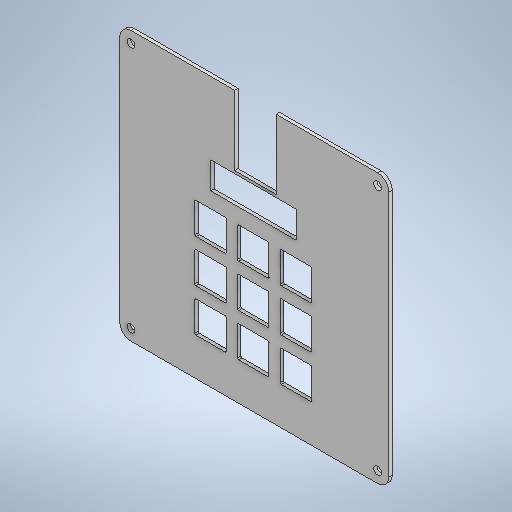
# Autodesk Inventor part: Top_Case_New
Saved by Autodesk Inventor 2025.1 (Build 291241000, 241)
## iProperties
Created: 2025-12-17
Part Number: Top_Case_New
Material: Generic
Document SubType Name: Modeling
Designer: omara
Density: 1 g/cm^3
Appearance: Default
Autodesk Inventor part; units mm, degrees
ref_plane "YZ Plane" through (0, 0, 0) normal (1, 0, 0) x (0, 1, 0)
ref_plane "XZ Plane" through (0, 0, 0) normal (0, 1, 0) x (-1, 0, 0)
ref_plane "XY Plane" through (0, 0, 0) normal (0, 0, 1) x (1, 0, 0)
sketch "Sketch1" plane through (0, 0, 0) normal (0, 0, 1) x (1, 0, 0)
  point P0 (0, 0)
sketch "0" plane through (0, 0, 0) normal (0, 0, 1) x (1, 0, 0)
  line L0 (3.025, -2.525) -> (16.025, -2.525)
  line L1 (3.025, -16.525) -> (16.025, -16.525)
  line L2 (2.525, -3.025) -> (2.525, -16.025)
  line L3 (16.525, -3.025) -> (16.525, -16.025)
  arc A0 (3.025, -2.525) -> (2.525, -3.025) centre (3.025, -3.025) ccw
  arc A1 (16.525, -3.025) -> (16.025, -2.525) centre (16.025, -3.025) ccw
  arc A2 (2.525, -16.025) -> (3.025, -16.525) centre (3.025, -16.025) ccw
  arc A3 (16.025, -16.525) -> (16.525, -16.025) centre (16.025, -16.025) ccw
  line L4 (22.075, -2.525) -> (35.075, -2.525)
  line L5 (22.075, -16.525) -> (35.075, -16.525)
  line L6 (21.575, -3.025) -> (21.575, -16.025)
  line L7 (35.575, -3.025) -> (35.575, -16.025)
  arc A4 (22.075, -2.525) -> (21.575, -3.025) centre (22.075, -3.025) ccw
  arc A5 (35.575, -3.025) -> (35.075, -2.525) centre (35.075, -3.025) ccw
  arc A6 (21.575, -16.025) -> (22.075, -16.525) centre (22.075, -16.025) ccw
  arc A7 (35.075, -16.525) -> (35.575, -16.025) centre (35.075, -16.025) ccw
  line L8 (41.125, -2.525) -> (54.125, -2.525)
  line L9 (41.125, -16.525) -> (54.125, -16.525)
  line L10 (40.625, -3.025) -> (40.625, -16.025)
  line L11 (54.625, -3.025) -> (54.625, -16.025)
  arc A8 (41.125, -2.525) -> (40.625, -3.025) centre (41.125, -3.025) ccw
  arc A9 (54.625, -3.025) -> (54.125, -2.525) centre (54.125, -3.025) ccw
  arc A10 (40.625, -16.025) -> (41.125, -16.525) centre (41.125, -16.025) ccw
  arc A11 (54.125, -16.525) -> (54.625, -16.025) centre (54.125, -16.025) ccw
  line L12 (3.025, -21.575) -> (16.025, -21.575)
  line L13 (3.025, -35.575) -> (16.025, -35.575)
  line L14 (2.525, -22.075) -> (2.525, -35.075)
  line L15 (16.525, -22.075) -> (16.525, -35.075)
  arc A12 (3.025, -21.575) -> (2.525, -22.075) centre (3.025, -22.075) ccw
  arc A13 (16.525, -22.075) -> (16.025, -21.575) centre (16.025, -22.075) ccw
  arc A14 (2.525, -35.075) -> (3.025, -35.575) centre (3.025, -35.075) ccw
  arc A15 (16.025, -35.575) -> (16.525, -35.075) centre (16.025, -35.075) ccw
  line L16 (22.075, -21.575) -> (35.075, -21.575)
  line L17 (22.075, -35.575) -> (35.075, -35.575)
  line L18 (21.575, -22.075) -> (21.575, -35.075)
  line L19 (35.575, -22.075) -> (35.575, -35.075)
  arc A16 (22.075, -21.575) -> (21.575, -22.075) centre (22.075, -22.075) ccw
  arc A17 (35.575, -22.075) -> (35.075, -21.575) centre (35.075, -22.075) ccw
  arc A18 (21.575, -35.075) -> (22.075, -35.575) centre (22.075, -35.075) ccw
  arc A19 (35.075, -35.575) -> (35.575, -35.075) centre (35.075, -35.075) ccw
  line L20 (41.125, -21.575) -> (54.125, -21.575)
  line L21 (41.125, -35.575) -> (54.125, -35.575)
  line L22 (40.625, -22.075) -> (40.625, -35.075)
  line L23 (54.625, -22.075) -> (54.625, -35.075)
  arc A20 (41.125, -21.575) -> (40.625, -22.075) centre (41.125, -22.075) ccw
  arc A21 (54.625, -22.075) -> (54.125, -21.575) centre (54.125, -22.075) ccw
  arc A22 (40.625, -35.075) -> (41.125, -35.575) centre (41.125, -35.075) ccw
  arc A23 (54.125, -35.575) -> (54.625, -35.075) centre (54.125, -35.075) ccw
  line L24 (3.025, -40.625) -> (16.025, -40.625)
  line L25 (3.025, -54.625) -> (16.025, -54.625)
  line L26 (2.525, -41.125) -> (2.525, -54.125)
  line L27 (16.525, -41.125) -> (16.525, -54.125)
  arc A24 (3.025, -40.625) -> (2.525, -41.125) centre (3.025, -41.125) ccw
  arc A25 (16.525, -41.125) -> (16.025, -40.625) centre (16.025, -41.125) ccw
  arc A26 (2.525, -54.125) -> (3.025, -54.625) centre (3.025, -54.125) ccw
  arc A27 (16.025, -54.625) -> (16.525, -54.125) centre (16.025, -54.125) ccw
  line L28 (22.075, -40.625) -> (35.075, -40.625)
  line L29 (22.075, -54.625) -> (35.075, -54.625)
  line L30 (21.575, -41.125) -> (21.575, -54.125)
  line L31 (35.575, -41.125) -> (35.575, -54.125)
  arc A28 (22.075, -40.625) -> (21.575, -41.125) centre (22.075, -41.125) ccw
  arc A29 (35.575, -41.125) -> (35.075, -40.625) centre (35.075, -41.125) ccw
  arc A30 (21.575, -54.125) -> (22.075, -54.625) centre (22.075, -54.125) ccw
  arc A31 (35.075, -54.625) -> (35.575, -54.125) centre (35.075, -54.125) ccw
  line L32 (41.125, -40.625) -> (54.125, -40.625)
  line L33 (41.125, -54.625) -> (54.125, -54.625)
  line L34 (40.625, -41.125) -> (40.625, -54.125)
  line L35 (54.625, -41.125) -> (54.625, -54.125)
  arc A32 (41.125, -40.625) -> (40.625, -41.125) centre (41.125, -41.125) ccw
  arc A33 (54.625, -41.125) -> (54.125, -40.625) centre (54.125, -41.125) ccw
  arc A34 (40.625, -54.125) -> (41.125, -54.625) centre (41.125, -54.125) ccw
  arc A35 (54.125, -54.625) -> (54.625, -54.125) centre (54.125, -54.125) ccw
  line L36 (-30.946, 48.585) -> (89.054, 48.585)
  line L37 (89.054, 48.585) -> (89.054, -71.415)
  line L38 (89.054, -71.415) -> (-30.946, -71.415)
  line L39 (-30.946, -71.415) -> (-30.946, 48.585)
  line L40 (20.309, 48.585) -> (38.809, 48.585)
  line L41 (38.809, 48.585) -> (38.809, 17.585)
  line L42 (38.809, 17.585) -> (20.309, 17.585)
  line L43 (20.309, 17.585) -> (20.309, 48.585)
  circle A36 centre (-25.946, 43.585) radius 1.7
  circle A37 centre (84.054, 43.585) radius 1.7
  circle A38 centre (84.054, -66.415) radius 1.7
  circle A39 centre (-25.946, -66.415) radius 1.7
  line L44 (9.675, 16.395) -> (47.675, 16.395)
  line L45 (47.675, 16.395) -> (47.675, 4.395)
  line L46 (47.675, 4.395) -> (9.675, 4.395)
  line L47 (9.675, 4.395) -> (9.675, 16.395)
  point P0 (9.525, -54.625)
  dimension "d0" = 120
  dimension "d1" = 120
  dimension "d2" = 33.471
  dimension "d3" = 16.79
  dimension "d4" = 18.5
  dimension "d5" = 31
  dimension "d6" = 51.255
  dimension "d7" = 3.4
  dimension "d8" = 3.4
  dimension "d9" = 3.4
  dimension "d10" = 3.4
  dimension "d11" = 5
  dimension "d12" = 5
  dimension "d13" = 5
  dimension "d14" = 5
  dimension "d15" = 5
  dimension "d16" = 5
  dimension "d17" = 5
  dimension "d18" = 5
  dimension "d19" = 38
  dimension "d20" = 12
  dimension "d21" = 40.621
  dimension "d22" = 32.19
  constraints: 96 end point, 72 point on circle, 40 centre point, 21 horizontal, 18 vertical, 6 parallel, 3 perpendicular, 1 midpoint, 1 point on line, 216 other
  measures "d0" distance of L37.end L38.end
  measures "d1" distance of L36.end L37.end
  measures "d2" distance between parallel lines of L39 L26
  measures "d3" distance from line of L38 point (9.525, -54.625)
  measures "d4" distance of L41.end L42.end
  measures "d5" distance of L40.end L41.end
  measures "d6" distance between parallel lines of L39 L43
  measures "d7" diameter of A36
  measures "d8" diameter of A37
  measures "d9" diameter of A38
  measures "d10" diameter of A39
  measures "d11" distance from line of L38 A39.centre
  measures "d12" distance from line of A39.centre L39
  measures "d13" distance from line of L37 A38.centre
  measures "d14" distance from line of L38 A38.centre
  measures "d15" distance from line of L37 A37.centre
  measures "d16" distance from line of L36 A37.centre
  measures "d17" distance from line of L36 A36.centre
  measures "d18" distance from line of L39 A36.centre
  measures "d19" distance of L45.end L46.end
  measures "d20" distance of L44.end L45.end
  measures "d21" distance between parallel lines of L39 L47
  measures "d22" distance between parallel lines of L36 L44
extrude "Extrusion1" add sketch "0" along normal blind 1.5 contours L36 L43 L42 L41 L37 L38 L39
fillet "Fillet1" radius 5 4 edges at (-30.946, -71.415, 0.75) (89.054, -71.415, 0.75) (89.054, 48.585, 0.75) (-30.946, 48.585, 0.75)
body "Solid1"
